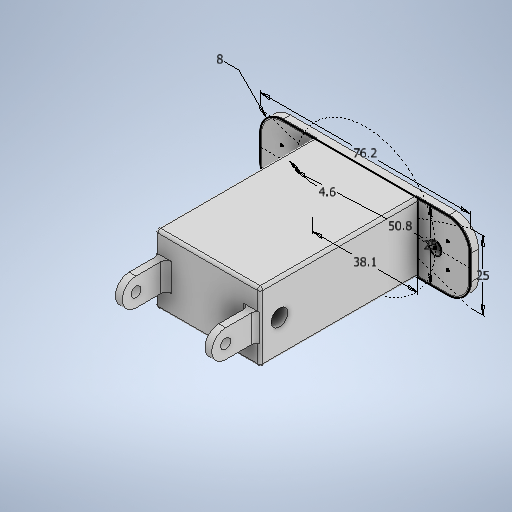
# Autodesk Inventor part: camstand2.25inch tallWithEarsForCam
Saved by Autodesk Inventor 2025 (Build 290162000, 162)
## iProperties
Created: 2025-03-15
Part Number: camstand2.25inch tallWithEarsForCam
Material: Generic
Document SubType Name: Modeling
Designer: john
Density: 1 g/cm^3
Appearance: Default
Author: john
Autodesk Inventor part; units mm, degrees
ref_plane "YZ Plane" through (0, 0, 0) normal (1, 0, 0) x (0, 1, 0)
ref_plane "XZ Plane" through (0, 0, 0) normal (0, 1, 0) x (-1, 0, 0)
ref_plane "XY Plane" through (0, 0, 0) normal (0, 0, 1) x (1, 0, 0)
sketch "Sketch1" plane through (0, 0, 0) normal (0, 0, 1) x (1, 0, 0)
  line L0 (-30.1, -12.5) -> (30.1, -12.5)
  line L1 (38.1, -4.5) -> (38.1, 4.5)
  line L2 (30.1, 12.5) -> (-30.1, 12.5)
  line L3 (-38.1, 4.5) -> (-38.1, -4.5)
  line L4 (-38.1, -12.5) -> (38.1, 12.5) construction
  line L5 (38.1, -12.5) -> (-38.1, 12.5) construction
  line L6 (-38.1, 0) -> (38.1, 0) construction
  line L7 (0, 12.5) -> (0, -12.5) construction
  circle A0 centre (0, 0) radius 25.4 construction
  line L8 (-19.05, 12.5) -> (19.05, 12.5) construction
  line L9 (19.05, 12.5) -> (19.05, -12.5)
  line L10 (19.05, -12.5) -> (-19.05, -12.5) construction
  line L11 (-19.05, -12.5) -> (-19.05, 12.5)
  line L12 (-19.05, 12.5) -> (19.05, -12.5) construction
  line L13 (19.05, 12.5) -> (-19.05, -12.5) construction
  circle A1 centre (-25.4, 0) radius 2.3
  circle A2 centre (25.4, 0) radius 2.3
  arc A3 (-30.1, 12.5) -> (-38.1, 4.5) centre (-30.1, 4.5) ccw
  arc A4 (-38.1, -4.5) -> (-30.1, -12.5) centre (-30.1, -4.5) ccw
  arc A5 (30.1, -12.5) -> (38.1, -4.5) centre (30.1, -4.5) ccw
  arc A6 (38.1, 4.5) -> (30.1, 12.5) centre (30.1, 4.5) ccw
  dimension "d2" = 50.8
  dimension "d0" = 76.2
  dimension "d1" = 25
  dimension "d3" = 38.1
  dimension "d4" = 25
  dimension "d5" = 4.6
  dimension "d6" = 8
  constraints: 28 end point, 9 point on line, 8 midpoint, 8 point on circle, 8 tangent, 6 centre point, 4 parallel, 3 equal radius, 2 horizontal, 2 perpendicular, 1 coincident, 1 horizontal alignment, 1 symmetric about line, 3 other
  measures "d0" distance of L5.end L4.end
  measures "d1" distance of L4.end L5.start
  measures "d3" distance of L9.end L10.end
  measures "d4" distance of L8.end L9.end
  measures "d5" diameter of A1
  measures "d6" radius of A3
extrude "Extrusion1" add sketch "Sketch1" against normal blind 3
extrude "Extrusion2" add sketch "Sketch1" along normal blind 57.15 contours L11 L2 L9 L0
sketch "Sketch2" plane through (19.05, -12.5, 0) normal (1, 0, 0) x (0, 0, -1)
  line L0 (-57.15, 0) -> (-57.15, 25) construction
  line L1 (-57.15, 12.5) -> (3, 12.5) construction
  line L2 (3, 8) -> (3, 17) construction
  circle A0 centre (-50.15, 12.5) radius 3
  point P0 (0, 12.5)
  dimension "d11" = 6
  dimension "d12" = 7
  constraints: 2 end point, 2 midpoint, 1 centre point, 1 point on line
  measures "d11" diameter of A0
  measures "d12" distance from line of A0.centre L0
extrude "Extrusion3" cut sketch "Sketch2" against normal blind 44.45
fillet "Fillet1" radius 1 4 edges at (19.05, -12.5, 28.575) (19.05, 12.5, 28.575) (-19.05, 12.5, 28.575) (-19.05, -12.5, 28.575)
fillet "Fillet2" radius 1 8 edges at (-18.7571, -12.2071, 57.15) (0, -12.5, 57.15) (18.7571, -12.2071, 57.15) (19.05, 0, 57.15) (18.7571, 12.2071, 57.15) (0, 12.5, 57.15) (-18.7571, 12.2071, 57.15) (-19.05, 0, 57.15)
fillet "Fillet3" radius 0.5 14 edges at (-35.7569, -10.1569, 0) (-18.55, -12.5, 0) (-24.575, -12.5, 0) (-35.7569, 10.1569, 0) (-18.55, 12.5, 0) (-24.575, 12.5, 0) (-38.1, 0, 0) (38.1, 0, 0) (35.7569, 10.1569, 0) (18.55, 12.5, 0) (24.575, 12.5, 0) (18.55, -12.5, 0) (24.575, -12.5, 0) (35.7569, -10.1569, 0)
sketch "Sketch3" plane through (0, 0, 57.15) normal (0, 0, 1) x (1, 0, 0)
  line L0 (15, 5) -> (15, -5)
  line L1 (-15, -5) -> (-15, 5)
  line L2 (-15, 5) -> (15, -5) construction
  line L3 (15, 5) -> (-15, -5) construction
  line L4 (-15, 5) -> (-17.5, 5)
  line L5 (-17.5, 5) -> (-17.5, -5)
  line L6 (-17.5, -5) -> (-15, -5)
  line L7 (17.5, 5) -> (15, 5)
  line L8 (15, -5) -> (17.5, -5)
  line L9 (17.5, 5) -> (17.5, -5)
  line L10 (18.05, 11.5) -> (18.05, -11.5) projected
  point P0 (0, 0)
  dimension "d18" = 30
  dimension "d19" = 10
  dimension "d20" = 2.5
  dimension "d21" = 2.5
  constraints: 20 end point, 2 horizontal, 2 midpoint, 2 parallel, 2 perpendicular
  measures "d18" distance of L0.end L1.start
  measures "d19" distance of L0.start L0.end
  measures "d20" distance of L1.end L4.end
  measures "d21" distance of L7.start L7.end
extrude "Extrusion4" add sketch "Sketch3" along normal blind 16
fillet "Fillet4" radius 2 4 edges at (-15, 0, 57.15) (15, 0, 57.15) (17.5, 0, 57.15) (-17.5, 0, 57.15)
fillet "Fillet5" radius 5 4 edges at (-16.25, -5, 73.15) (-16.25, 5, 73.15) (16.25, 5, 73.15) (16.25, -5, 73.15)
sketch "Sketch4" plane through (-17.5, -5, 58.7763) normal (-1, 0, 0) x (0, 0, 1)
  line L0 (0, 10) -> (9.3737, 10) construction
  line L1 (9.3737, 10) -> (9.3737, 0.0421) construction
  circle A0 centre (9.3737, 5.0211) radius 1.8
  point P0 (-58.7763, 5)
  dimension "d26" = 3.6
  constraints: 2 end point, 1 centre point, 1 midpoint, 1 vertical
  measures "d26" diameter of A0
extrude "Extrusion5" cut sketch "Sketch4" against normal blind 55
body "Solid1"
